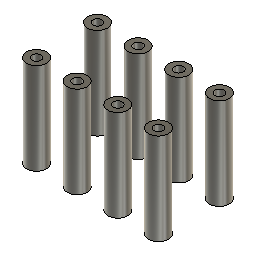
Pin 30mm v1 (Autodesk Fusion 360 design; units mm, degrees)
Autodesk Fusion 360 part; units mm, degrees
sketch "Sketch1" plane through (0, 0, 0) normal (0, 0, 1) x (1, 0, 0)
  circle A0 centre (0, 0) radius 3.25
  dimension "d1" = 6.5
  constraint coincident A0.centre origin
  measures "d1" diameter of A0
extrude "Extrude1" add sketch "Sketch1" along normal blind 30 makes body 1
sketch "Sketch2" plane through (0, 0, 30) normal (0, 0, 1) x (-1, 0, 0)
  circle A0 centre (0, 0) radius 3.25
  circle A1 centre (0, 0) radius 1.49
  dimension "d4" = 2.98
  constraint coincident A0.centre A1.centre
  measures "d4" diameter of A1
extrude "Extrude2" cut sketch "Sketch2" against normal blind 30 contours A1 bodies 1
pattern_linear "R-Pattern1" count 4 spacing 13.3333 along (1, 0, 0) count 2 spacing 20 along (0, 1, 0) of "Extrude1", "Extrude2" makes body 2 at (16.5672, -0.3236, 20) makes body 3 at (29.9005, -0.3236, 20) makes body 4 at (43.2339, -0.3236, 20) makes body 5 at (3.2339, 19.6764, 20) makes body 6 at (16.5672, 19.6764, 20) makes body 7 at (29.9005, 19.6764, 20) makes body 8 at (43.2339, 19.6764, 20)
